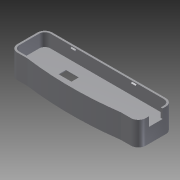
# Autodesk Inventor part: case_front
Saved by Autodesk Inventor 2014 (Build 180170000, 170)
## iProperties
Created: 2013-11-09
Part Number: case_front
Material: Generic
Document SubType Name: Modeling
Designer: Tyler
Density: 1 g/cm^3
Appearance: Default
Author: Tyler
Autodesk Inventor part; units mm, degrees
ref_plane "YZ Plane" through (0, 0, 0) normal (1, 0, 0) x (0, 1, 0)
ref_plane "XZ Plane" through (0, 0, 0) normal (0, 1, 0) x (-1, 0, 0)
ref_plane "XY Plane" through (0, 0, 0) normal (0, 0, 1) x (1, 0, 0)
sketch "Sketch1" plane through (0, 0, 0) normal (0, 0, 1) x (1, 0, 0)
  line L0 (-62, 19) -> (62, 19)
  line L1 (70, 11) -> (70, -11)
  line L2 (62, -19) -> (-62, -19)
  line L3 (-70, -11) -> (-70, 11)
  arc A0 (-62, 19) -> (-70, 11) centre (-62, 11) ccw
  arc A1 (-70, -11) -> (-62, -19) centre (-62, -11) ccw
  arc A2 (70, 11) -> (62, 19) centre (62, 11) ccw
  arc A3 (62, -19) -> (70, -11) centre (62, -11) ccw
  point P0 (0, 0)
  point P1 (70, -19)
  point P2 (70, 19)
  point P3 (-70, -19)
  dimension "d0" = 140
  dimension "d1" = 38
  dimension "d2" = 70
  dimension "d3" = 19
  dimension "d4" = 8
  dimension "d5" = 8
  dimension "d6" = 8
  dimension "d7" = 8
  constraints: 8 end point, 8 point on circle, 8 tangent, 6 point on line, 4 centre point, 2 parallel, 1 horizontal, 1 perpendicular
  measures "d0" distance of point (70, -19) point (-70, -19)
  measures "d1" distance of point (70, 19) point (70, -19)
  measures "d2" distance from line of L3 point (0, 0)
  measures "d3" distance from line of L2 point (0, 0)
  measures "d4" radius of A0
  measures "d5" radius of A1
  measures "d6" radius of A2
  measures "d7" radius of A3
extrude "Extrusion1" add sketch "Sketch1" against normal blind 15
sketch "Sketch2" plane through (0, 0, 0) normal (0, 0, 1) x (1, 0, 0)
  line L0 (-62, 19) -> (62, 19) projected
  arc A0 (-62, 19) -> (-70, 11) centre (-62, 11) ccw projected
  line L1 (-70, -11) -> (-70, 11) projected
  arc A1 (-70, -11) -> (-62, -19) centre (-62, -11) ccw projected
  line L2 (62, -19) -> (-62, -19) projected
  arc A2 (62, -19) -> (70, -11) centre (62, -11) ccw projected
  line L3 (70, 11) -> (70, -11) projected
  arc A3 (70, 11) -> (62, 19) centre (62, 11) ccw projected
  line L4 (62, 17) -> (-62, 17)
  arc A4 (-62, 17) -> (-68, 11) centre (-62, 11) ccw
  line L5 (-68, 11) -> (-68, -11)
  arc A5 (-68, -11) -> (-62, -17) centre (-62, -11) ccw
  line L6 (-62, -17) -> (62, -17)
  arc A6 (62, -17) -> (68, -11) centre (62, -11) ccw
  line L7 (68, -11) -> (68, 11)
  arc A7 (68, 11) -> (62, 17) centre (62, 11) ccw
  point P0 (0, 0)
  dimension "d10" = 2
  constraints: 8 end point, 8 point on circle, 4 centre point, 7 other
  measures "d10" distance between parallel lines of L4 L0
extrude "Extrusion2" cut sketch "Sketch2" against normal blind 14 contours A7 L7 A6 L6 A5 L5 A4 L4
sketch "Sketch3" plane through (70, -11, 0) normal (1, 0, 0) x (0, 0, -1)
  line L0 (0, 22) -> (0, 0) projected
  line L1 (-6.9158, 18.5) -> (10, 18.5)
  line L2 (10, 18.5) -> (10, 3.5)
  line L3 (10, 3.5) -> (-6.9158, 3.5)
  line L4 (-6.9158, 3.5) -> (-6.9158, 18.5)
  point P0 (0, 11)
  dimension "d13" = 6.9158
  dimension "d14" = 10
  dimension "d15" = 15
  dimension "d16" = 7.5
  constraints: 8 end point, 2 parallel, 1 horizontal, 1 perpendicular
  measures "d13" distance between parallel lines of L4 L0
  measures "d14" distance between parallel lines of L2 L0
  measures "d15" distance of L1.end L2.end
  measures "d16" distance from line of L3 point (0, 11)
extrude "Extrusion3" cut sketch "Sketch3" against normal blind 14
sketch "Sketch4" plane through (0, 0, -14) normal (0, 0, 1) x (1, 0, 0)
  line L0 (-62, -17) -> (62, -17) projected
  line L1 (62, 17) -> (-62, 17) projected
  line L2 (27, 19) -> (32, 19)
  line L3 (32, 19) -> (32, 16)
  line L4 (32, 16) -> (27, 16)
  line L5 (27, 16) -> (27, 19)
  line L6 (32, -19) -> (27, -19)
  line L7 (27, -19) -> (27, -16)
  line L8 (27, -16) -> (32, -16)
  line L9 (32, -16) -> (32, -19)
  line L10 (-42, -19) -> (-47, -19)
  line L11 (-47, -19) -> (-47, -16)
  line L12 (-47, -16) -> (-42, -16)
  line L13 (-42, -16) -> (-42, -19)
  line L14 (70, 7.5) -> (70, -7.5) projected
  line L15 (62, -19) -> (-62, -19) projected
  line L16 (-62, 19) -> (62, 19) projected
  line L17 (-39, 19) -> (-34, 19)
  line L18 (-34, 19) -> (-34, 16)
  line L19 (-34, 16) -> (-39, 16)
  line L20 (-39, 16) -> (-39, 19)
  line L21 (-70, -11) -> (-70, 11) projected
  point P0 (0, 0)
  dimension "d19" = 38
  dimension "d20" = 5
  dimension "d21" = 5
  dimension "d22" = 38
  dimension "d23" = 1
  dimension "d24" = 1
  dimension "d25" = 0
  dimension "d26" = 0
  dimension "d28" = 1
  dimension "d29" = 0
  dimension "d30" = 5
  dimension "d31" = 5
  dimension "d33" = 1
  dimension "d34" = 0
  dimension "d59" = 66
  dimension "d60" = 74
  constraints: 32 end point, 8 parallel, 4 horizontal, 4 perpendicular
  measures "d19" distance from line of L6.start L14
  measures "d20" distance between parallel lines of L9 L7
  measures "d21" distance between parallel lines of L5 L3
  measures "d22" distance between parallel lines of L14 L3
  measures "d23" distance between parallel lines of L4 L1
  measures "d24" distance between parallel lines of L0 L8
  measures "d25" distance between parallel lines of L15 L6
  measures "d26" distance between parallel lines of L16 L2
  measures "d28" distance between parallel lines of L19 L1
  measures "d29" distance between parallel lines of L16 L17
  measures "d30" distance of L18.end L19.end
  measures "d31" distance of L11.end L12.end
  measures "d33" distance between parallel lines of L0 L12
  measures "d34" distance between parallel lines of L15 L10
  measures "d59" distance of L3.end L18.end
  measures "d60" distance between parallel lines of L9 L13
extrude "Extrusion4" add sketch "Sketch4" along normal blind 13 contours L11 L12 L13 L0 | L0 L13 L10 L11 | L7 L8 L9 L0 | L0 L9 L6 L7 | L3 L4 L5 L1 | L1 L5 L2 L3 | L18 L19 L20 L1 | L1 L20 L16 L18
chamfer "Chamfer1" distance 1 distance2 1 1 edges at (-36.5, 16, -1) measured on face at (-36.5, 16, -1.5)
chamfer "Chamfer3" distance 1 distance2 1 1 edges at (29.5, 16, -1) measured on face at (29.5, 16, -1.5)
chamfer "Chamfer4" distance 1 distance2 1 1 edges at (-44.5, -16, -1) measured on face at (-44.5, -16, -1.5)
chamfer "Chamfer5" distance 1 distance2 1 1 edges at (29.5, -16, -1) measured on face at (29.5, -16, -1.5)
sketch "Sketch5" plane through (0, 0, -14) normal (0, 0, 1) x (1, 0, 0)
  line L0 (-39, 17) -> (-62, 17) projected
  arc A0 (-62, 17) -> (-68, 11) centre (-62, 11) ccw projected
  line L1 (-68, 11) -> (-68, -11) projected
  arc A1 (-68, -11) -> (-62, -17) centre (-62, -11) ccw projected
  line L2 (-62, -17) -> (-47, -17) projected
  line L3 (-47, -17) -> (-47, -16) projected
  line L4 (-47, -16) -> (-42, -16) projected
  line L5 (-42, -16) -> (-42, -17) projected
  line L6 (-42, -17) -> (27, -17) projected
  line L7 (27, -17) -> (27, -16) projected
  line L8 (27, -16) -> (32, -16) projected
  line L9 (32, -16) -> (32, -17) projected
  line L10 (32, -17) -> (62, -17) projected
  line L11 (-49, 17) -> (37, 17)
  line L12 (37, 17) -> (37, -17)
  line L13 (37, -17) -> (-49, -17)
  line L14 (-49, -17) -> (-49, 17)
  point P0 (32, 16)
  point P1 (-39, 16)
  point P2 (0, 0)
  dimension "d53" = 10
  dimension "d54" = 5
  constraints: 8 end point, 2 parallel, 2 point on line, 1 horizontal, 1 perpendicular
  measures "d53" distance from line of point (-39, 16) L14
  measures "d54" distance from line of point (32, 16) L12
extrude "Extrusion5" cut sketch "Sketch5" along normal blind 11
sketch "Sketch8" plane through (0, 0, 0) normal (0, 0, 1) x (1, 0, 0)
  line L0 (-70, -11) -> (-70, 11) projected
  line L1 (62, -19) -> (-62, -19) projected
  line L2 (70, -7.5) -> (70, -11) projected
  line L3 (62, -17) -> (-62, -17) projected
  line L4 (0, -22.5) -> (0, -17) construction
  arc A0 (-52, -18.8579) -> (52, -18.8579) centre (0, 350.5357) ccw
  arc A1 (-49.9899, -19.1353) -> (-52, -19) centre (-52, -34) ccw
  arc A2 (52, -19) -> (49.9899, -19.1353) centre (52, -34) ccw
  line L5 (-52, -19) -> (-52, -17)
  line L6 (52, -19) -> (52, -17)
  line L7 (52, -17) -> (-52, -17)
  point P0 (0, 0)
  dimension "d63" = 2
  dimension "d64" = 18
  dimension "d65" = 18
  dimension "d66" = 5.5
  dimension "d67" = 30
  dimension "d68" = 30
  constraints: 9 point on circle, 8 end point, 6 point on line, 4 tangent, 3 centre point, 3 perpendicular, 1 collinear, 1 midpoint
  measures "d63" distance between parallel lines of L1 L3
  measures "d64" distance from line of L2 A2.centre
  measures "d65" distance from line of A1.centre L0
  measures "d66" distance of L4.start L4.end
  measures "d67" diameter of A1
  measures "d68" diameter of A2
extrude "Extrusion8" add sketch "Sketch8" against normal up to surface (15 mm away) contours A0 L1 | L1 A0 L5 L3 L6
sketch "Sketch11" plane through (0, 0, -14) normal (0, 0, 1) x (1, 0, 0)
  line L0 (62, 17) -> (-62, 17) projected
  line L1 (-68, 11) -> (-68, -11) projected
  line L2 (-33, 5) -> (-19, 5)
  line L3 (-19, 5) -> (-19, -8)
  line L4 (-19, -8) -> (-33, -8)
  line L5 (-33, -8) -> (-33, 5)
  point P0 (0, 0)
  dimension "d78" = 35
  dimension "d79" = 14
  dimension "d80" = 12
  dimension "d81" = 13
  constraints: 8 end point, 2 parallel, 1 horizontal, 1 perpendicular
  measures "d78" distance between parallel lines of L1 L5
  measures "d79" distance of L2.start L2.end
  measures "d80" distance between parallel lines of L0 L2
  measures "d81" distance of L2.end L3.end
extrude "Extrusion10" cut sketch "Sketch11" against normal blind 10
sketch "Sketch12" plane through (0, 0, -15) normal (0, 0, -1) x (-1, 0, 0)
  line L0 (62, -19) -> (50.9804, -19) projected
  arc A0 (62, -19) -> (70, -11) centre (62, -11) ccw projected
  line L1 (70, 11) -> (70, -11) projected
  arc A1 (70, 11) -> (62, 19) centre (62, 11) ccw projected
  line L2 (-62, 19) -> (62, 19) projected
  arc A2 (-62, 19) -> (-70, 11) centre (-62, 11) ccw projected
  line L3 (-70, -11) -> (-70, 11) projected
  arc A3 (-70, -11) -> (-62, -19) centre (-62, -11) ccw projected
  line L4 (-50.9804, -19) -> (-62, -19) projected
  arc A4 (-50.9804, -19) -> (50.9804, -19) centre (0, 350.5357) ccw projected
  arc A5 (67, 11) -> (62, 16) centre (62, 11) ccw
  line L5 (67, 11) -> (67, -11)
  arc A6 (62, -16) -> (67, -11) centre (62, -11) ccw
  line L6 (62, -16) -> (50.774, -16)
  arc A7 (-50.774, -16) -> (50.774, -16) centre (0, 350.5357) ccw
  line L7 (-50.774, -16) -> (-62, -16)
  arc A8 (-67, -11) -> (-62, -16) centre (-62, -11) ccw
  line L8 (-67, -11) -> (-67, 11)
  arc A9 (-62, 16) -> (-67, 11) centre (-62, 11) ccw
  line L9 (-62, 16) -> (62, 16)
  point P0 (0, 0)
  dimension "d84" = 3
  constraints: 10 end point, 10 point on circle, 5 centre point, 9 other
  measures "d84" distance between parallel lines of L9 L2
extrude "Extrusion11" add sketch "Sketch12" along normal blind 10
lip "Lip1" kind lip height 1 width 1 edges at (0, 19, -25) (67.6569, 16.6569, -25) (70, 0, -25) (67.6569, -16.6569, -25) (56.4902, -19, -25) (-67.6569, 16.6569, -25) (-70, 0, -25) (-67.6569, -16.6569, -25) (-56.4902, -19, -25) (0, -22.5, -25) guide face at (20.6667, 18, -25)
sketch "Sketch13" plane through (0, 0, -15) normal (0, 0, -1) x (-1, 0, 0)
  line L0 (67, -11) -> (67, 11) projected
  line L1 (-67, 11) -> (-67, -11) projected
  line L2 (-67, -9.1) -> (67, -9.1)
  line L3 (67, -9.1) -> (67, -11.1)
  line L4 (67, -11.1) -> (-67, -11.1)
  line L5 (-67, -11.1) -> (-67, -9.1)
  line L6 (-62, -19) -> (-50.9804, -19) projected
  point P0 (0, 0)
  dimension "d93" = 2
  dimension "d95" = 9.9
  dimension "d96" = 0
  dimension "d97" = 0
  constraints: 8 end point, 2 parallel, 1 horizontal, 1 perpendicular
  measures "d93" distance between parallel lines of L4 L2
  measures "d95" distance between parallel lines of L2 L6
  measures "d96" distance between parallel lines of L1 L5
  measures "d97" distance between parallel lines of L0 L3
extrude "Extrusion12" add sketch "Sketch13" along normal blind 2
sketch "Sketch14" plane through (0, 0, -17) normal (0, 0, -1) x (-1, 0, 0)
  line L0 (-66.999, -11.1) -> (66.999, -11.1) projected
  line L1 (-64.26, -9.1) -> (-62.26, -9.1)
  line L2 (-62.26, -9.1) -> (-62.26, -11.1)
  line L3 (-62.26, -11.1) -> (-67, -11.1)
  line L4 (-67, -11.1) -> (-67, -9.1)
  line L5 (-70, 11) -> (-70, -11) projected
  line L6 (67, -9.1) -> (-67, -9.1) projected
  line L7 (-64.26, -5.1) -> (-67, -5.1)
  line L8 (-67, -5.1) -> (-67, -9.1)
  line L9 (-64.26, -9.1) -> (-64.26, -5.1)
  point P0 (0, 0)
  dimension "d103" = 7.74
  dimension "d104" = 2
  dimension "d106" = 4
  dimension "d107" = 2
  constraints: 14 end point, 3 parallel, 2 horizontal, 2 perpendicular, 1 point on line
  measures "d103" distance between parallel lines of L5 L2
  measures "d104" distance between parallel lines of L2 L9
  measures "d106" distance between parallel lines of L6 L7
  measures "d107" distance between parallel lines of L0 L1
extrude "Extrusion13" add sketch "Sketch14" against normal blind 2 and the other way blind 8
equation "\"d2\" = 0.5 * d0"
equation "\"d3\" = 0.5 * d1"
equation "\"d16\" = 0.5 * d15"
body "Solid1"
